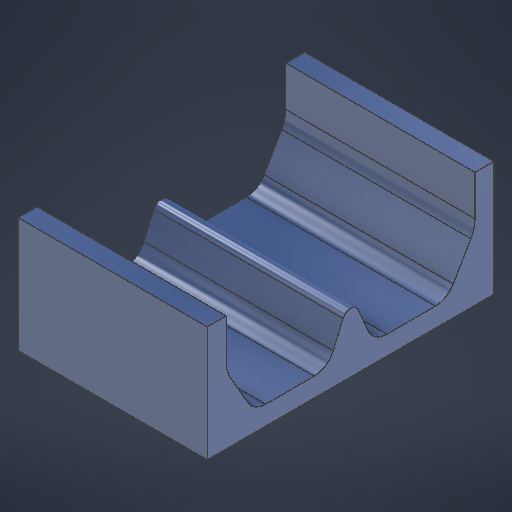
# Autodesk Inventor part: wago_support
Saved by Autodesk Inventor 2026.1 (Build 301233000, 233)
## iProperties
Created: 2026-04-25
Part Number: wago_support
Material: Generic
Document SubType Name: Modeling
Designer: emanuel
Density: 1 g/cm^3
Appearance: Default
Author: emanuel
Autodesk Inventor part; units mm, degrees
ref_plane "YZ Plane" through (0, 0, 0) normal (1, 0, 0) x (0, 1, 0)
ref_plane "XZ Plane" through (0, 0, 0) normal (0, 1, 0) x (-1, 0, 0)
ref_plane "XY Plane" through (0, 0, 0) normal (0, 0, 1) x (1, 0, 0)
sketch "Sketch1" plane through (0, 0, 0) normal (1, 0, 0) x (0, 1, 0)
  arc A0 (-7.974, 10.8816) -> (-8.874, 9.3228) centre (-7.074, 9.3228) ccw
  line L0 (-8.874, 9.3228) -> (-8.874, 3.4133)
  line L1 (-8.874, 9.3228) -> (-8.874, 3.4133)
  arc A1 (-1.981, -0.7039) -> (0, -1) centre (-0.4181, 2.9781) ccw
  line L2 (-7.7773, 1.7564) -> (-1.981, -0.7039)
  line L3 (2.1178, 13.4219) -> (-2.7701, 13.4219)
  line L4 (-1.981, -0.7039) -> (2.1178, 13.4219)
  line L5 (2.1178, 13.4219) -> (-2.7701, 13.4219)
  arc A2 (-2.7701, 13.4219) -> (-4.2701, 13.02) centre (-2.7701, 10.4219) ccw
  line L6 (-4.2701, 13.02) -> (-12.9304, 8.02)
  line L7 (-4.2701, 13.02) -> (-7.974, 10.8816)
  circle A3 centre (-7.074, 9.3228) radius 1.8
  circle A4 centre (-2.7701, 10.4219) radius 3
  arc A5 (-8.874, 3.4133) -> (-7.7773, 1.7564) centre (-7.074, 3.4133) ccw
  circle A6 centre (-7.074, 3.4133) radius 1.8
  line L8 (0, -1) -> (-3.8233, -1)
  arc A7 (-8.874, -11.3228) -> (-7.974, -12.8816) centre (-7.074, -11.3228) ccw
  line L9 (-8.874, -11.3228) -> (-8.874, -5.4133)
  line L10 (-8.874, -11.3228) -> (-8.874, -5.4133)
  line L11 (-7.7773, -3.7564) -> (-1.981, -1.2961)
  line L12 (2.1178, -15.4219) -> (-2.7701, -15.4219)
  line L13 (-1.981, -1.2961) -> (2.1178, -15.4219)
  line L14 (2.1178, -15.4219) -> (-2.7701, -15.4219)
  arc A8 (-4.2701, -15.02) -> (-2.7701, -15.4219) centre (-2.7701, -12.4219) ccw
  line L15 (-4.2701, -15.02) -> (-12.9304, -10.02)
  line L16 (-4.2701, -15.02) -> (-7.974, -12.8816)
  circle A9 centre (-7.074, -11.3228) radius 1.8
  circle A10 centre (-2.7701, -12.4219) radius 3
  arc A11 (-7.7773, -3.7564) -> (-8.874, -5.4133) centre (-7.074, -5.4133) ccw
  circle A12 centre (-7.074, -5.4133) radius 1.8
  line L17 (-1.981, -0.7039) -> (-1.981, -1.2961)
  line L18 (2.1178, 13.4219) -> (2.1178, 16.4219)
  line L19 (2.1178, 16.4219) -> (-11.8822, 16.4219)
  line L20 (-11.8822, 16.4219) -> (-11.8822, -18.4221)
  line L21 (-11.8822, -18.4221) -> (2.1178, -18.4221)
  line L22 (2.1178, -18.4221) -> (2.1178, -15.4219)
  point P0 (0, 0)
  point P1 (4.8736, 0.62)
  point P2 (-0.4181, -4.9781)
  point P3 (-4.2701, -15.02)
  point P4 (-7.974, 10.8816)
  dimension "d0" = 10
  dimension "d1" = 3
  dimension "d2" = 14
  dimension "d3" = 34.844
  constraints: 46 end point, 16 symmetric about line, 14 point on circle, 11 centre point, 6 coincident, 4 perpendicular, 3 collinear, 2 horizontal, 2 vertical, 1 point on line, 1 tangent, 1 vertical alignment, 10 other
  measures "d0" distance of L6.start L6.end
  measures "d1" distance of L3.start L18.end
  measures "d2" distance of L18.end L19.end
  measures "d3" distance of L19.end L20.end
extrude "Extrusion1" add sketch "Sketch1" along normal blind 23 contours L6 L20 L19 L18 L3 A2 | A0 L0 A5 L2 L17 L11 A11 L9 A7 L15 L20 L6 | L15 A8 L12 L22 L21 L20
sketch "Sketch2" plane through (23, 0, 0) normal (1, 0, 0) x (0, 0, -1)
  line L0 (-13.4219, -2.7701) -> (-13.4219, 2.1178) projected
  line L1 (-13.4219, 2.1178) -> (-13.4219, -2.7701)
  line L2 (-13.4219, -2.7701) -> (-14.1219, -2.7701)
  line L3 (-14.1219, -2.7701) -> (-14.1219, 2.1178)
  line L4 (-14.1219, 2.1178) -> (-13.4219, 2.1178)
  line L5 (-10.8816, -7.974) -> (-13.02, -4.2701) projected
  line L6 (-13.02, -4.2701) -> (-10.8816, -7.974)
  line L7 (-10.8816, -7.974) -> (-11.4878, -8.324)
  line L8 (-11.4878, -8.324) -> (-13.6262, -4.6201)
  line L9 (-13.6262, -4.6201) -> (-13.02, -4.2701)
  arc A0 (-10.8816, -7.974) -> (-9.3228, -8.874) centre (-9.3228, -7.074) ccw projected
  arc A1 (-3.4133, -8.874) -> (-1.7564, -7.7773) centre (-3.4133, -7.074) ccw projected
  line L10 (-9.3228, -8.874) -> (-3.4133, -8.874)
  line L11 (-3.4133, -8.874) -> (-3.4133, -9.574)
  line L12 (-3.4133, -9.574) -> (-9.3228, -9.574)
  line L13 (-9.3228, -9.574) -> (-9.3228, -8.874)
  line L14 (0.7039, -1.981) -> (-1.7564, -7.7773) projected
  line L15 (-1.7564, -7.7773) -> (0.7039, -1.981)
  line L16 (0.7039, -1.981) -> (1.3483, -2.2546)
  line L17 (1.3483, -2.2546) -> (-1.1121, -8.0508)
  line L18 (-1.1121, -8.0508) -> (-1.7564, -7.7773)
  line L19 (1.2961, -1.981) -> (0.7039, -1.981) projected
  line L20 (1, -1.981) -> (1, -3.9334)
  arc A2 (-13.4219, -2.7701) -> (-13.02, -4.2701) centre (-10.4219, -2.7701) ccw projected
  circle A3 centre (-10.4219, -2.7701) radius 3.7
  circle A4 centre (-9.3228, -7.074) radius 2.5
  circle A5 centre (-3.4133, -7.074) radius 2.5
  line L21 (15.4219, -2.7701) -> (15.4219, 2.1178)
  line L22 (15.4219, 2.1178) -> (15.4219, -2.7701)
  line L23 (15.4219, -2.7701) -> (16.1219, -2.7701)
  line L24 (16.1219, -2.7701) -> (16.1219, 2.1178)
  line L25 (16.1219, 2.1178) -> (15.4219, 2.1178)
  line L26 (12.8816, -7.974) -> (15.02, -4.2701)
  line L27 (15.02, -4.2701) -> (12.8816, -7.974)
  line L28 (12.8816, -7.974) -> (13.4878, -8.324)
  line L29 (13.4878, -8.324) -> (15.6262, -4.6201)
  line L30 (15.6262, -4.6201) -> (15.02, -4.2701)
  arc A6 (11.3228, -8.874) -> (12.8816, -7.974) centre (11.3228, -7.074) ccw
  arc A7 (3.7564, -7.7773) -> (5.4133, -8.874) centre (5.4133, -7.074) ccw
  line L31 (11.3228, -8.874) -> (5.4133, -8.874)
  line L32 (5.4133, -8.874) -> (5.4133, -9.574)
  line L33 (5.4133, -9.574) -> (11.3228, -9.574)
  line L34 (11.3228, -9.574) -> (11.3228, -8.874)
  line L35 (1.2961, -1.981) -> (3.7564, -7.7773)
  line L36 (3.7564, -7.7773) -> (1.2961, -1.981)
  line L37 (0.6517, -2.2546) -> (3.1121, -8.0508)
  line L38 (3.1121, -8.0508) -> (3.7564, -7.7773)
  arc A8 (15.02, -4.2701) -> (15.4219, -2.7701) centre (12.4219, -2.7701) ccw
  circle A9 centre (12.4219, -2.7701) radius 3.7
  circle A10 centre (11.3228, -7.074) radius 2.5
  circle A11 centre (5.4133, -7.074) radius 2.5
  point P0 (0, 0)
  point P1 (13.7491, -6.4715)
  point P2 (13.6826, -6.2487)
  point P3 (13.9372, -6.1456)
  point P4 (-11.9372, -6.1456)
  point P5 (-11.6826, -6.2487)
  point P6 (-11.7491, -6.4715)
  point P7 (-13.6262, -4.6201)
  point P8 (-9.3228, -9.574)
  point P9 (-1.1121, -8.0508)
  point P10 (1, -3.0751)
  point P11 (3.1121, -8.0508)
  point P12 (11.3228, -9.574)
  point P13 (15.6262, -4.6201)
  point P14 (16.1219, -2.7701)
  point P15 (15.4219, -0.6045)
  point P16 (9.6476, -5.2182)
  point P17 (9.5878, -8.874)
  point P18 (7.1483, -8.874)
  point P19 (3.0785, -6.1803)
  point P20 (-1.0785, -6.1803)
  point P21 (-5.1483, -8.874)
  point P22 (-7.5878, -8.874)
  point P23 (-7.6476, -5.2182)
  point P24 (-13.4219, -0.6045)
  point P25 (-14.1219, -2.7701)
  dimension "d6" = 0.7
  dimension "d7" = 0.7
  dimension "d8" = 0.7
  dimension "d9" = 0.7
  constraints: 70 end point, 21 symmetric about line, 9 parallel, 6 coincident, 6 point on circle, 5 centre point, 4 perpendicular, 3 collinear, 3 vertical, 2 tangent, 1 midpoint, 16 other
  measures "d6" distance of L0.start L2.end
  measures "d7" distance of L5.start L7.end
  measures "d8" distance of L10.end L11.end
  measures "d9" distance of L14.start L16.end
extrude "Extrusion2" cut sketch "Sketch2" against normal blind 23 contours L2 A3 L0 | A2 L9 A3 L2 | L0 A3 A4 L5 A2 | A3 L3 L4 L0 | L5 A3 L9 | A3 L5 A4 L8 | A4 L10 A0 L5 A3 | A3 A4 | A4 L5 L7 | L7 A0 L13 A4 | A4 L10 A5 L12 | L13 L10 A4 | A5 L10 L11 | L11 A1 L18 A5 | A5 L14 A1 L10 | A5 L14 L16 L20 L17 | L18 L14 A5 | L20 L16 L17 | L17 L16 L20 L19 L35 A11 L37 | L19 L20 L16 | A11 L35 L38 | L38 A7 L32 A11 | L35 A11 L31 A7 | A11 L31 A10 L33 | L32 L31 A11 | A10 L31 L34 | L34 A6 L28 A10 | L31 A10 A9 L26 A6 | A10 L26 A9 L29 | L28 L26 A10 | A9 L26 L30 | L30 A8 L23 A9 | A10 A9 | A9 L21 A8 L26 A10 | A9 L21 L25 L24 | L23 L21 A9
fillet "Fillet1" radius 1 1 edges at (11.5, -3.0751, -1)
body "Solid1"
